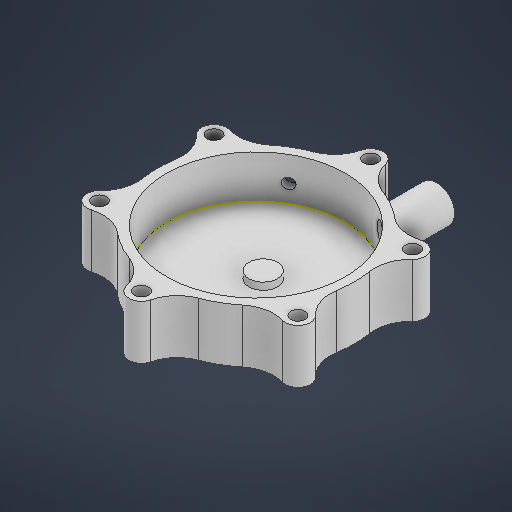
# Autodesk Inventor part: carcaza motor
Saved by Autodesk Inventor 2025.3 (Build 293356000, 356)
## iProperties
Created: 2025-10-02
Part Number: carcaza motor
Material: Generic
Document SubType Name: Modeling
Designer: sophi
Density: 1 g/cm^3
Appearance: Default
Author: sophi
Autodesk Inventor part; units mm, degrees
ref_plane "YZ Plane" through (0, 0, 0) normal (1, 0, 0) x (0, 1, 0)
ref_plane "XZ Plane" through (0, 0, 0) normal (0, 1, 0) x (-1, 0, 0)
ref_plane "XY Plane" through (0, 0, 0) normal (0, 0, 1) x (1, 0, 0)
sketch "Sketch1" plane through (0, 0, 0) normal (0, 1, 0) x (-1, 0, 0)
  circle A0 centre (0, 0) radius 27.5
  circle A1 centre (0, 0) radius 25
  circle A2 centre (0, -32) radius 3.5
  arc A3 (9.6311, -25.7583) -> (3.4049, -32.8102) centre (13.1333, -35.125) ccw
  line L0 (0, -39.6745) -> (0, -15.9391) construction
  arc A4 (-3.4049, -32.8102) -> (-9.6311, -25.7583) centre (-13.1333, -35.125) ccw
  line L1 (47.8103, 0) -> (-62.0389, 0) construction
  circle A5 centre (0, -32) radius 2
  circle A6 centre (27.7128, -16) radius 3.5
  circle A7 centre (27.7128, -16) radius 2
  arc A8 (26.712, -19.3539) -> (17.4918, -21.22) centre (23.8525, -28.9363) ccw
  arc A9 (27.1229, -4.5384) -> (30.1169, -13.4563) centre (36.9858, -6.1887) ccw
  circle A10 centre (27.7128, 16) radius 3.5
  circle A11 centre (27.7128, 16) radius 2
  arc A12 (30.1169, 13.4563) -> (27.1229, 4.5384) centre (36.9858, 6.1887) ccw
  arc A13 (17.4918, 21.22) -> (26.712, 19.3539) centre (23.8525, 28.9363) ccw
  circle A14 centre (0, 32) radius 3.5
  circle A15 centre (0, 32) radius 2
  arc A16 (3.4049, 32.8102) -> (9.6311, 25.7583) centre (13.1333, 35.125) ccw
  arc A17 (-9.6311, 25.7583) -> (-3.4049, 32.8102) centre (-13.1333, 35.125) ccw
  circle A18 centre (-27.7128, 16) radius 3.5
  circle A19 centre (-27.7128, 16) radius 2
  arc A20 (-26.712, 19.3539) -> (-17.4918, 21.22) centre (-23.8525, 28.9363) ccw
  arc A21 (-27.1229, 4.5384) -> (-30.1169, 13.4563) centre (-36.9858, 6.1887) ccw
  circle A22 centre (-27.7128, -16) radius 3.5
  circle A23 centre (-27.7128, -16) radius 2
  arc A24 (-30.1169, -13.4563) -> (-27.1229, -4.5384) centre (-36.9858, -6.1887) ccw
  arc A25 (-17.4918, -21.22) -> (-26.712, -19.3539) centre (-23.8525, -28.9363) ccw
  point P0 (27.1229, 4.5384)
  point P1 (30.1169, 13.4563)
  point P2 (17.4918, 21.22)
  point P3 (9.6311, 25.7583)
  point P4 (3.4049, 32.8102)
  point P5 (-17.4918, 21.22)
  point P6 (-26.712, 19.3539)
  point P7 (-27.1229, 4.5384)
  point P8 (-27.1229, -4.5384)
  point P9 (-30.1169, -13.4563)
  point P10 (-9.6311, -25.7583)
  point P11 (-3.4049, -32.8102)
  point P12 (26.712, -19.3539)
  point P13 (27.1229, -4.5384)
  dimension "d16" = 55
  dimension "d18" = 7
  dimension "d17" = 50
  dimension "d19" = 32
  dimension "d21" = 10
  dimension "d22" = 4
  dimension "d25" = 360
  constraints: 24 point on circle, 19 centre point, 8 coincident, 4 end point, 3 symmetric about line, 2 point on line, 1 horizontal, 1 vertical, 1 vertical alignment, 97 other
  measures "d17" diameter of A1
  measures "d19" distance of point (0, 0) point (0, -32)
  measures "d21" radius of A3
  measures "d22" diameter of A5
extrude "Extrusion5" add sketch "Sketch1" along normal blind 15
extrude "Extrusion6" add sketch "Sketch1" along normal blind 3 contours A1
sketch "Sketch4" plane through (0, 3, 0) normal (0, 1, 0) x (1, 0, 0)
  circle A0 centre (0, 0) radius 25 projected
ref_plane "Work Plane3" through (0, 15, -35.5) normal (0, 0, -1) x (-1, 0, 0)
sketch "Sketch5" plane through (0, 15, -35.5) normal (0, 0, -1) x (-1, 0, 0)
  line L0 (-9.6311, -15) -> (-17.4918, -15) projected
  line L1 (-9.6311, 0) -> (-17.4918, 0) projected
  circle A0 centre (-15, -5) radius 5
  circle A1 centre (-15, -5) radius 3
  line L2 (3.4049, -15) -> (-3.4049, -15) projected
  circle A2 centre (20.2025, -6) radius 1.5
  point P0 (0, -15)
  point P1 (0, -15)
  dimension "d33" = 10
  dimension "d34" = 6
  dimension "d35" = 5
  dimension "d36" = 15
  dimension "d41" = 3
  constraints: 3 centre point, 1 coincident, 1 midpoint
  measures "d33" diameter of A0
  measures "d34" diameter of A1
  measures "d35" distance from line of L1 A0.centre
  measures "d36" horizontal distance of point (0, -15) A0.centre
  measures "d41" diameter of A2
extrude "Extrusion7" add sketch "Sketch5" against normal up to surface contours A0 | A1 round surface about axis through (0, 0, 0) along (0, 1, 0) radius 25 far side no
extrude "Extrusion8" cut sketch "Sketch5" against normal up to surface contours A1 round surface about axis through (0, 0, 0) along (0, 1, 0) radius 25 far side no
ref_plane "Work Plane4" through (-13.75, 15, -23.8157) normal (-0.5, 0, -0.8660254) x (0, -1, 0)
sketch "Sketch6" plane through (-13.75, 15, -23.8157) normal (-0.5, 0, -0.8660254) x (0, -1, 0)
  circle A0 centre (7, 0) radius 1.5
  line L0 (15, 4.5384) -> (15, -4.5384) projected
  point P0 (15, 0)
  point P1 (15, 0)
  point P2 (15, 0)
  dimension "d42" = 3
  dimension "d43" = 8
  constraints: 2 midpoint, 1 centre point, 1 horizontal alignment
  measures "d42" diameter of A0
  measures "d43" distance of point (15, 0) A0.centre
extrude "Extrusion9" cut sketch "Sketch6" against normal up to surface round surface about axis through (0, 0, 0) along (0, 1, 0) radius 25 far side no
sketch "Sketch8" plane through (0, 3, 0) normal (0, 1, 0) x (1, 0, 0)
  circle A0 centre (2, 0) radius 4
  circle A1 centre (2, 0) radius 22.5
  circle A2 centre (0, 0) radius 25 projected
  dimension "d50" = 8
  dimension "d51" = 45
  dimension "d52" = 2
  constraints: 2 centre point, 2 horizontal alignment, 1 concentric
  measures "d50" diameter of A0
  measures "d51" diameter of A1
  measures "d52" distance of A1.centre A2.centre
extrude "Extrusion11" add sketch "Sketch8" along normal blind 2 contours A0
body "Solid2"
